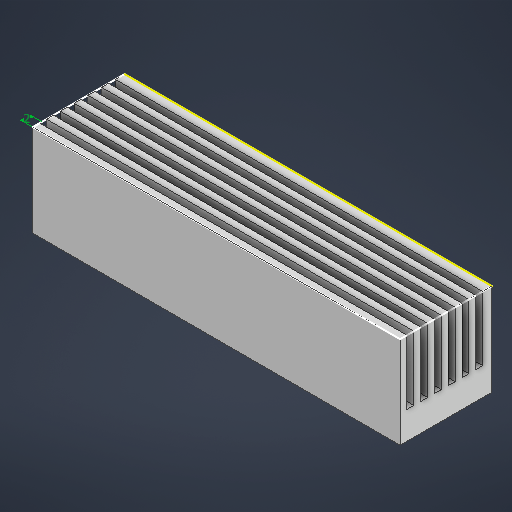
# Autodesk Inventor part: heatsink
Saved by Autodesk Inventor 2027.1 (Build 311270010, 270A)
## iProperties
Created: 2026-10-02
Part Number: heatsink
Material: Generic
Document SubType Name: Modeling
Designer: Arik
Density: 1 g/cm^3
Appearance: Default
Author: Arik
Autodesk Inventor part; units mm, degrees
ref_plane "YZ Plane" through (0, 0, 0) normal (1, 0, 0) x (0, 1, 0)
ref_plane "XZ Plane" through (0, 0, 0) normal (0, 1, 0) x (-1, 0, 0)
ref_plane "XY Plane" through (0, 0, 0) normal (0, 0, 1) x (1, 0, 0)
sketch "Sketch1" plane through (0, 0, 0) normal (0, 1, 0) x (-1, 0, 0)
  line L0 (0, 0) -> (80, 0)
  line L1 (80, 0) -> (80, -20)
  line L2 (80, -20) -> (0, -20)
  line L3 (0, -20) -> (0, 0)
  dimension "d0" = 80
  dimension "d1" = 20
  constraints: 8 end point, 2 parallel, 1 horizontal, 1 perpendicular
  measures "d0" distance of L1.end L2.end
  measures "d1" distance of L0.end L1.end
extrude "Extrusion1" add sketch "Sketch1" along normal blind 20
sketch "Sketch2" plane through (0, 20, 0) normal (0, 1, 0) x (1, 0, 0)
  line L0 (0, 20) -> (-80, 20) projected
  line L1 (0, 0) -> (-80, 0)
  line L2 (-80, 0) -> (-80, 20)
  line L3 (-80, 20) -> (0, 20)
  line L4 (0, 20) -> (0, 0)
  line L5 (-80, 0) -> (-80, 2)
  dimension "d4" = 2
  constraints: 10 end point, 2 parallel, 1 horizontal, 1 perpendicular, 1 point on line
  measures "d4" distance of L1.end L5.end
sketch "Sketch3" plane through (0, 20, 0) normal (0, 1, 0) x (1, 0, 0)
  line L0 (-80, 0) -> (0, 0) projected
  line L1 (0, 0) -> (-80, 0)
  line L2 (-80, 0) -> (-80, 1.5)
  line L3 (-80, 1.5) -> (0, 1.5)
  line L4 (0, 1.5) -> (0, 0)
  line L5 (0, 1.5) -> (-80, 1.5)
  line L6 (-80, 1.5) -> (-80, 3)
  line L7 (-80, 3) -> (0, 3)
  line L8 (0, 3) -> (0, 1.5)
  line L9 (0, 3) -> (-80, 3)
  line L10 (-80, 3) -> (-80, 4.5)
  line L11 (-80, 4.5) -> (0, 4.5)
  line L12 (0, 4.5) -> (0, 3)
  line L13 (0, 4.5) -> (-80, 4.5)
  line L14 (-80, 4.5) -> (-80, 6)
  line L15 (-80, 6) -> (0, 6)
  line L16 (0, 6) -> (0, 4.5)
  line L17 (0, 6) -> (-80, 6)
  line L18 (-80, 6) -> (-80, 7.5)
  line L19 (-80, 7.5) -> (0, 7.5)
  line L20 (0, 7.5) -> (0, 6)
  line L21 (0, 7.5) -> (-80, 7.5)
  line L22 (-80, 7.5) -> (-80, 9)
  line L23 (-80, 9) -> (0, 9)
  line L24 (0, 9) -> (0, 7.5)
  line L25 (0, 9) -> (-80, 9)
  line L26 (-80, 9) -> (-80, 10.5)
  line L27 (-80, 10.5) -> (0, 10.5)
  line L28 (0, 10.5) -> (0, 9)
  line L29 (0, 10.5) -> (-80, 10.5)
  line L30 (-80, 10.5) -> (-80, 12)
  line L31 (-80, 12) -> (0, 12)
  line L32 (0, 12) -> (0, 10.5)
  line L33 (0, 12) -> (-80, 12)
  line L34 (-80, 12) -> (-80, 13.5)
  line L35 (-80, 13.5) -> (0, 13.5)
  line L36 (0, 13.5) -> (0, 12)
  line L37 (0, 13.5) -> (-80, 13.5)
  line L38 (-80, 13.5) -> (-80, 15)
  line L39 (-80, 15) -> (0, 15)
  line L40 (0, 15) -> (0, 13.5)
  line L41 (0, 15) -> (-80, 15)
  line L42 (-80, 15) -> (-80, 16.5)
  line L43 (-80, 16.5) -> (0, 16.5)
  line L44 (0, 16.5) -> (0, 15)
  line L45 (0, 16.5) -> (-80, 16.5)
  line L46 (-80, 16.5) -> (-80, 18)
  line L47 (-80, 18) -> (0, 18)
  line L48 (0, 18) -> (0, 16.5)
  line L49 (0, 18) -> (-80, 18)
  line L50 (-80, 18) -> (-80, 19.5)
  line L51 (-80, 19.5) -> (0, 19.5)
  line L52 (0, 19.5) -> (0, 18)
  dimension "d5" = 80
  dimension "d6" = 1.5
  dimension "d7" = 80
  dimension "d8" = 1.5
  dimension "d9" = 80
  dimension "d10" = 1.5
  dimension "d11" = 80
  dimension "d12" = 1.5
  dimension "d13" = 80
  dimension "d14" = 1.5
  dimension "d15" = 80
  dimension "d16" = 1.5
  dimension "d17" = 80
  dimension "d18" = 1.5
  dimension "d19" = 80
  dimension "d20" = 1.5
  dimension "d21" = 80
  dimension "d22" = 1.5
  dimension "d23" = 80
  dimension "d24" = 1.5
  dimension "d25" = 80
  dimension "d26" = 1.5
  dimension "d27" = 80
  dimension "d28" = 1.5
  dimension "d29" = 80
  dimension "d30" = 1.5
  constraints: 104 end point, 26 parallel, 13 horizontal, 13 perpendicular
  measures "d5" distance of L2.end L3.end
  measures "d6" distance of L1.end L2.end
  measures "d7" distance of L6.end L7.end
  measures "d8" distance of L5.end L6.end
  measures "d9" distance of L10.end L11.end
  measures "d10" distance of L9.end L10.end
  measures "d11" distance of L14.end L15.end
  measures "d12" distance of L13.end L14.end
  measures "d13" distance of L18.end L19.end
  measures "d14" distance of L17.end L18.end
  measures "d15" distance of L22.end L23.end
  measures "d16" distance of L21.end L22.end
  measures "d17" distance of L26.end L27.end
  measures "d18" distance of L25.end L26.end
  measures "d19" distance of L30.end L31.end
  measures "d20" distance of L29.end L30.end
  measures "d21" distance of L34.end L35.end
  measures "d22" distance of L33.end L34.end
  measures "d23" distance of L38.end L39.end
  measures "d24" distance of L37.end L38.end
  measures "d25" distance of L42.end L43.end
  measures "d26" distance of L41.end L42.end
  measures "d27" distance of L46.end L47.end
  measures "d28" distance of L45.end L46.end
  measures "d29" distance of L50.end L51.end
  measures "d30" distance of L49.end L50.end
extrude "Extrusion2" cut sketch "Sketch3" against normal blind 14 contours L6 L7 L8 L3 | L14 L15 L16 L11 | L22 L23 L24 L19 | L30 L31 L32 L27 | L38 L39 L40 L35 | L46 L47 L48 L43
body "Solid1"
